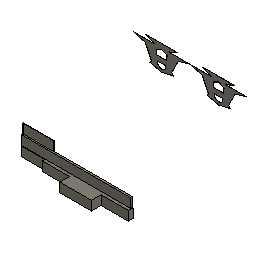
final drawing i hope v4 (Autodesk Fusion 360 design; units mm, degrees)
Autodesk Fusion 360 part; units mm, degrees
note: some values were not read from the file. Chosen so that the rebuilt part matches the saved one: which bodies a step acts on.
sketch "Sketch2" plane through (0, 0, 0) normal (0, 0, 1) x (1, 0, 0)
  line L0 (0, 0) -> (2438.4, 0)
  line L1 (2438.4, 0) -> (2438.4, 1219.2)
  line L2 (2438.4, 1219.2) -> (0, 1219.2)
  line L3 (0, 1219.2) -> (0, 0)
  line L4 (542.8322, 1080.4856) -> (1889.3565, 1080.4856)
  line L5 (1889.3565, 1080.4856) -> (1510.789, 917.945)
  line L6 (1510.789, 917.945) -> (2425.5578, 917.945)
  line L7 (2425.5578, 917.945) -> (1919.9959, 772.756)
  line L8 (1919.9959, 772.756) -> (1642.7832, 207.6244)
  line L9 (1642.7832, 207.6244) -> (1722.6773, 131.0438)
  line L10 (1722.6773, 131.0438) -> (1213.6665, 11.8411)
  line L11 (1211.4478, 868.4674) -> (1211.4478, 1080.4856)
  line L12 (1211.4478, 1080.4856) -> (1213.6665, 11.8411)
  line L13 (1213.6665, 11.8411) -> (1213.6665, 0)
  line L14 (1213.6665, 130.0044) -> (1361.4547, 188.3424)
  line L15 (1361.4547, 188.3424) -> (1391.2443, 341.6348)
  line L16 (1391.2443, 341.6348) -> (1212.9825, 341.2647)
  line L17 (1212.5359, 556.3863) -> (1420.4572, 556.818)
  line L18 (1420.4572, 556.818) -> (1446.4012, 750.0109)
  line L19 (1446.4012, 750.0109) -> (1211.4478, 868.4674)
  line L20 (1213.6665, 130.0044) -> (1361.4547, 188.3424)
  line L21 (1391.2443, 341.6348) -> (1361.4547, 188.3424)
  line L22 (1212.9825, 341.2647) -> (1391.2443, 341.6348)
  line L23 (1215.082, 130.5632) -> (1213.4213, 129.9077)
  dimension "d1" = 2438.4
  dimension "d2" = 1219.2
  constraint horizontal L0
  constraint vertical L1
  constraint horizontal L2
  constraint vertical L3
  constraint coincident L0.start L3.end
  constraint horizontal L4
  constraint perpendicular L1 L6
  constraint coincident L4 L11.end
  constraint perpendicular L4 L11
  constraint coincident L0 L13.end
  constraint perpendicular L0 L13
  constraint coincident L12 L16.end
  constraint perpendicular L12 L16
  constraint coincident L12 L17.start
  constraint perpendicular L12 L17
  constraint coincident L14 L23.start
  constraint coincident L12 L23.end
  constraint parallel L14 L23
  measures "d1" distance of L0.start L0.end
  measures "d2" distance of L0.start L2.end
extrude "Extrude1" add sketch "Sketch2" along normal blind 3.175 contours L4 L5 L6 L7 L8 L9 L10 L12 L14 L15 L16 L17 L18 L19 L20 L21 L22 L23 makes body 1
extrude "Extrude2" add 1 faces at (1661.0788, 512.3995, 3.175) along direction (0, 0, 1) blind 3.175 on bodies 1 bodies 1
mirror "Mirror1" about plane through (1212.5359, 556.3863, 0) normal (-0.999998, -0.002076, 0) of bodies 1 merged
sketch "Sketch3" plane through (0, 0, 0) normal (0, 0, 1) x (1, 0, 0)
  line L0 (0, 0) -> (-609.6, 0)
  line L1 (-609.6, 0) -> (-609.6, 406.4)
  line L2 (-609.6, 406.4) -> (0, 406.4)
  line L3 (0, 406.4) -> (0, 0)
  dimension "d9" = 609.6
  dimension "d10" = 406.4
  constraint horizontal L0
  constraint vertical L1
  constraint horizontal L2
  constraint vertical L3
  constraint coincident L0.start L3.end
  measures "d9" distance of L0.start L0.end
  measures "d10" distance of L0.start L2.end
scale "Scale1" factor 0.25 about (1004.6146, 555.9546, 6.35) bodies 1
move_body "Move1" bodies 1 to x (1, 0, 0) y (0, 1, 0) z (0, 0, 1) at (-1360.9962, -410.5353, 0)
scale "Scale2" factor 0.99 about (-356.3816, 145.4193, 6.35) bodies 1
move_body "Move2" bodies 1 to x (0, -1, 0) y (1, 0, 0) z (0, 0, 1) at (-608.2009, -92.7478, 0)
scale "Scale3" factor 0.650517 about (-332.9602, 212.4425, 4.7784) bodies 1
move_body "Move3" bodies 1 to x (1, 0, 0) y (0, 1, 0) z (0, 0, 1) at (-97.2386, -6.7841, 0)
sketch "Sketch4" plane through (0, 0, 0) normal (0, 1, 0) x (1, 0, 0)
sketch "Sketch5" plane through (0, 0, 0) normal (0, 0, 1) x (1, 0, 0)
  line L0 (203.9021, 0) -> (788.7117, 0)
  line L1 (788.7117, 196.85) -> (203.9021, 196.85)
  line L2 (203.9021, 196.85) -> (203.9021, 0)
  line L3 (203.9021, 0) -> (288.0777, 0)
  line L4 (288.0777, 0) -> (288.0777, 196.85)
  line L5 (288.0777, 196.85) -> (203.9021, 196.85)
  line L6 (203.9021, 196.85) -> (203.9021, 0)
  line L7 (288.0777, 196.85) -> (305.8831, 196.85)
  line L8 (305.8831, 196.85) -> (305.8831, 0)
  line L9 (305.8831, 0) -> (288.0777, 0)
  line L10 (288.0777, 0) -> (288.0777, 196.85)
  line L11 (305.8831, 196.85) -> (407.2291, 196.85)
  line L12 (407.2291, 196.85) -> (407.2291, 0)
  line L13 (407.2291, 0) -> (305.8831, 0)
  line L14 (305.8831, 0) -> (305.8831, 196.85)
  line L15 (407.2291, 196.85) -> (491.9127, 196.85)
  line L16 (491.9127, 196.85) -> (491.9127, 0)
  line L17 (491.9127, 0) -> (407.2291, 0)
  line L18 (407.2291, 0) -> (407.2291, 196.85)
  line L19 (491.9127, 196.85) -> (639.1819, 196.85)
  line L20 (639.1819, 196.85) -> (639.1819, 0)
  line L21 (639.1819, 0) -> (491.9127, 0)
  line L22 (491.9127, 0) -> (491.9127, 196.85)
  line L23 (639.1819, 196.85) -> (706.7713, 196.85)
  line L24 (706.7713, 196.85) -> (706.7713, 0)
  line L25 (706.7713, 0) -> (639.1819, 0)
  line L26 (639.1819, 0) -> (639.1819, 196.85)
  line L27 (706.7713, 196.85) -> (732.1713, 196.85)
  line L28 (732.1713, 196.85) -> (732.1713, 0)
  line L29 (732.1713, 0) -> (706.7713, 0)
  line L30 (706.7713, 0) -> (706.7713, 196.85)
  line L31 (732.1713, 196.85) -> (757.3173, 196.85)
  line L32 (757.3173, 196.85) -> (757.3173, 0)
  line L33 (757.3173, 0) -> (732.1713, 0)
  line L34 (732.1713, 0) -> (732.1713, 196.85)
  line L35 (757.3173, 196.85) -> (788.7117, 196.85)
  line L36 (788.7117, 196.85) -> (788.7117, 0)
  line L37 (788.7117, 0) -> (757.3173, 0)
  line L38 (757.3173, 0) -> (757.3173, 196.85)
  line L39 (203.9021, 98.425) -> (788.7117, 98.425)
  dimension "d15" = 196.85
  dimension "d16" = 84.1756
  dimension "d17" = 17.8054
  dimension "d18" = 101.346
  dimension "d19" = 84.6836
  dimension "d20" = 147.2692
  dimension "d21" = 67.5894
  dimension "d22" = 25.4
  dimension "d23" = 25.146
  dimension "d24" = 31.3944
  constraint horizontal L0
  constraint horizontal L1
  constraint vertical L2
  constraint horizontal L3
  constraint vertical L4
  constraint horizontal L5
  constraint vertical L6
  constraint coincident L1 L4.end
  constraint horizontal L7
  constraint vertical L8
  constraint horizontal L9
  constraint vertical L10
  constraint horizontal L11
  constraint vertical L12
  constraint horizontal L13
  constraint vertical L14
  constraint horizontal L15
  constraint vertical L16
  constraint horizontal L17
  constraint vertical L18
  constraint coincident L0 L16.end
  constraint horizontal L19
  constraint vertical L20
  constraint horizontal L21
  constraint vertical L22
  constraint horizontal L23
  constraint vertical L24
  constraint horizontal L25
  constraint vertical L26
  constraint coincident L0 L24.end
  constraint horizontal L27
  constraint vertical L28
  constraint horizontal L29
  constraint vertical L30
  constraint coincident L0 L28.end
  constraint horizontal L31
  constraint vertical L32
  constraint horizontal L33
  constraint vertical L34
  constraint horizontal L35
  constraint vertical L36
  constraint horizontal L37
  constraint vertical L38
  constraint midpoint L2 L39.start
  constraint midpoint L36 L39.end
  measures "d15" distance of L0.start L1.end
  measures "d16" distance of L0.start L3.end
  measures "d17" distance of L4.end L7.end
  measures "d18" distance of L7.end L11.end
  measures "d19" distance of L11.end L15.end
  measures "d20" distance of L15.end L19.end
  measures "d21" distance of L19.end L23.end
  measures "d22" distance of L23.end L27.end
  measures "d23" distance of L27.end L31.end
  measures "d24" distance of L31.end L1.start
sketch "Sketch6" plane through (0, 0, 0) normal (0, 0, 1) x (1, 0, 0)
  line L0 (822.2364, 571.8843) -> (212.6364, 571.8843)
  line L1 (212.6364, 571.8843) -> (212.6364, 375.0343)
  line L2 (212.6364, 375.0343) -> (822.2364, 375.0343)
  line L3 (822.2364, 375.0343) -> (822.2364, 571.8843)
  line L4 (212.6364, 571.8843) -> (254.9274, 571.8843)
  line L5 (254.9274, 571.8843) -> (254.9274, 375.0343)
  line L6 (254.9274, 375.0343) -> (212.6364, 375.0343)
  line L7 (212.6364, 375.0343) -> (212.6364, 571.8843)
  line L8 (254.9274, 571.8843) -> (312.3314, 571.8843)
  line L9 (312.3314, 571.8843) -> (312.3314, 473.4593)
  line L10 (312.3314, 375.0343) -> (254.9274, 375.0343)
  line L11 (254.9274, 375.0343) -> (254.9274, 571.8843)
  line L12 (212.6364, 473.4593) -> (254.9274, 473.4593)
  line L13 (312.3314, 571.8843) -> (379.2858, 571.8843)
  line L14 (379.2858, 571.8843) -> (379.2858, 473.4593)
  line L15 (379.2858, 375.0343) -> (312.3314, 375.0343)
  line L16 (312.3314, 473.4593) -> (312.3314, 571.8843)
  line L17 (254.9274, 473.4593) -> (379.2858, 473.4593)
  line L18 (254.9274, 473.4593) -> (473.215, 473.4593)
  line L19 (473.215, 473.4593) -> (473.215, 375.0343)
  line L20 (473.215, 375.0343) -> (254.9274, 375.0343)
  line L21 (254.9274, 375.0343) -> (254.9274, 473.4593)
  dimension "d25" = 609.6
  dimension "d26" = 196.85
  dimension "d27" = 42.291
  dimension "d28" = 57.404
  dimension "d29" = 66.9544
  dimension "d30" = 218.2876
  constraint horizontal L0
  constraint vertical L1
  constraint horizontal L2
  constraint vertical L3
  constraint horizontal L4
  constraint vertical L5
  constraint horizontal L6
  constraint vertical L7
  constraint horizontal L8
  constraint vertical L9
  constraint horizontal L10
  constraint vertical L11
  constraint coincident L2 L10.start
  constraint midpoint L7 L12.start
  constraint midpoint L11 L12.end
  constraint perpendicular L11 L12
  constraint horizontal L13
  constraint vertical L14
  constraint horizontal L15
  constraint vertical L16
  constraint coincident L2 L15.start
  constraint coincident L17 L9.end
  constraint horizontal L18
  constraint vertical L19
  constraint horizontal L20
  constraint vertical L21
  measures "d25" distance of L0.start L0.end
  measures "d26" distance of L0.start L2.end
  measures "d27" distance of L0.end L4.end
  measures "d28" distance of L4.end L8.end
  measures "d29" distance of L8.end L13.end
  measures "d30" distance of L12.end L18.end
extrude "Extrude3" add sketch "Sketch6" along normal blind 3.175 separate body contours L2 L5 L10 L11 L15 L17 L18 L19 L20 L21 makes body 2
move_body "Move4" bodies 2 to x (1, 0, 0) y (0, 1, 0) z (0, 0, 1) at (-384.6431, 161.5704, 0)
move_body "Move5" bodies 2 to x (0, -1, 0) y (0, 0, 1) z (-1, 0, 0) at (-430.0903, 185.4213, -530.8446)
extrude "Extrude4" add sketch "Sketch6" along normal blind 3.175 separate body contours L0 L9 L13 L14 L16 L17 L18 makes body 3
move_body "Move6" bodies 3 to x (0, -1, 0) y (0, 0, 1) z (-1, 0, 0) at (-514.5757, 550.6973, -468.49)
extrude "Extrude5" add sketch "Sketch6" along normal blind 3.175 separate body contours L0 L5 L8 L9 L11 L16 L17 L18 makes body 4
move_body "Move7" bodies 4 to x (0, 1, 0) y (0, 0, -1) z (-1, 0, 0) at (-545.9307, -77.9718, 577.731)
extrude "Extrude6" add sketch "Sketch6" along normal blind 3.175 separate body contours L0 L1 L4 L5 L7 L11 L12 makes body 5
move_body "Move8" bodies 5 to x (0.5, -0.866025, 0) y (0, 0, 1) z (-0.866025, -0.5, 0) at (-590.0447, 429.1998, -467.7351)
move_body "Move9" bodies 5 to x (0.99863, -0.052336, 0) y (0.052336, 0.99863, 0) z (0, 0, 1) at (-10.4106, -25.2848, 0)
copy_body "CopyPasteBodies1" bodies 5 makes body 6
move_body "Move10" bodies 6 to x (-0.587785, 0.809017, 0) y (-0.809017, -0.587785, 0) z (0, 0, 1) at (-568.0051, 700.1132, 0)
extrude "Extrude7" add sketch "Sketch5" along normal blind 3.175 separate body contours L1 L32 L35 L36 L38 L39 makes body 7
move_body "Move11" bodies 7 to x (0.990268, -0.139173, 0) y (0, 0, -1) z (0.139173, 0.990268, 0) at (-1264.9245, 274.1917, 98.425)
move_body "Move12" bodies 7 to x (1, 0, 0) y (0, 1, 0) z (0, 0, 1) at (0, 0, 104.14)
copy_body "CopyPasteBodies2" bodies 7 makes body 8
move_body "Move13" bodies 8 to x (0.956305, 0.292372, 0) y (-0.292372, 0.956305, 0) z (0, 0, 1) at (26.9574, 228.0991, 0)
scale "Scale4" factor 0.8 about (-514.8682, 238.9524, 5.715) bodies 1 7 4 5 2 6 3 8
sketch "Sketch7" plane through (0, 0, 0) normal (0, 0, 1) x (1, 0, 0)
  line L0 (0, 0) -> (196.85, 0)
  line L1 (196.85, 0) -> (196.85, 609.6)
  line L2 (196.85, 609.6) -> (0, 609.6)
  line L3 (0, 609.6) -> (0, 0)
  line L4 (0, 0) -> (98.425, 0)
  line L5 (98.425, 0) -> (98.425, 596.9)
  line L6 (98.425, 596.9) -> (0, 596.9)
  line L7 (0, 596.9) -> (0, 0)
  line L8 (0, 596.9) -> (196.85, 596.9)
  line L9 (196.85, 596.9) -> (196.85, 0)
  line L10 (196.85, 0) -> (0, 0)
  line L11 (0, 0) -> (0, 596.9)
  dimension "d42" = 196.85
  dimension "d43" = 609.6
  dimension "d44" = 98.425
  dimension "d45" = 596.9
  constraint horizontal L0
  constraint vertical L1
  constraint horizontal L2
  constraint vertical L3
  constraint coincident L0.start L3.end
  constraint horizontal L4
  constraint vertical L5
  constraint horizontal L6
  constraint vertical L7
  constraint horizontal L8
  constraint vertical L9
  constraint horizontal L10
  constraint vertical L11
  measures "d42" distance of L0.start L0.end
  measures "d43" distance of L0.start L2.end
  measures "d44" distance of L0.start L4.end
  measures "d45" distance of L0.start L6.end
sketch "Sketch8" plane through (0, 0, 0) normal (0, 0, 1) x (1, 0, 0)
  line L0 (-854.4402, -1.7894) -> (-1464.0402, -1.7894)
  line L1 (-1464.0402, -1.7894) -> (-1464.0402, 404.6106)
  line L2 (-1464.0402, 404.6106) -> (-854.4402, 404.6106)
  line L3 (-854.4402, 404.6106) -> (-854.4402, -1.7894)
  line L4 (-854.4402, 404.6106) -> (-1017.3075, 404.6106)
  line L5 (-1017.3075, 404.6106) -> (-1017.3075, 306.1856)
  line L6 (-1017.3075, 306.1856) -> (-854.4402, 306.1856)
  line L7 (-854.4402, 306.1856) -> (-854.4402, 404.6106)
  dimension "d46" = 609.6
  dimension "d47" = 406.4
  dimension "d48" = 162.8673
  dimension "d49" = 98.425
  constraint horizontal L0
  constraint vertical L1
  constraint horizontal L2
  constraint vertical L3
  constraint horizontal L4
  constraint vertical L5
  constraint horizontal L6
  constraint vertical L7
  measures "d46" distance of L0.start L0.end
  measures "d47" distance of L0.start L2.end
  measures "d48" distance of L2.end L4.end
  measures "d49" distance of L2.end L6.end
move_body "Move14" bodies 1 to x (1, 0, 0) y (0, 1, 0) z (0, 0, 1) at (-411.614, -53.3151, 0)
scale "Scale5" factor 0.869565 about (-981.0371, 93.1545, 4.9657) bodies 1
move_body "Move15" bodies 1 to x (1, 0, 0) y (0, 1, 0) z (0, 0, 1) at (15.801, -12.4151, 0)
sketch "Sketch9" plane through (0, 0, 0) normal (0, 0, 1) x (1, 0, 0)
  line L0 (-852.6405, 515.8905) -> (-852.6405, 319.0405)
  line L1 (-852.6405, 319.0405) -> (-1462.2405, 319.0405)
  line L2 (-1462.2405, 319.0405) -> (-1462.2405, 515.8905)
  line L3 (-1462.2405, 515.8905) -> (-852.6405, 515.8905)
  line L4 (-852.6405, 515.8905) -> (-852.6405, 417.4655)
  line L5 (-852.6405, 417.4655) -> (-1426.8837, 417.4655)
  line L6 (-1426.8837, 417.4655) -> (-1426.8837, 515.8905)
  line L7 (-1426.8837, 515.8905) -> (-852.6405, 515.8905)
  line L8 (-852.6405, 417.4655) -> (-852.6405, 319.0405)
  line L9 (-852.6405, 319.0405) -> (-1294.3465, 319.0405)
  line L10 (-1294.3465, 319.0405) -> (-1294.3465, 417.4655)
  line L11 (-1294.3465, 417.4655) -> (-852.6405, 417.4655)
  line L12 (-1462.2405, 319.0405) -> (-1462.2405, 417.4655)
  line L13 (-1462.2405, 417.4655) -> (-1337.8821, 417.4655)
  line L14 (-1337.8821, 417.4655) -> (-1337.8821, 319.0405)
  line L15 (-1337.8821, 319.0405) -> (-1462.2405, 319.0405)
  dimension "d51" = 196.85
  dimension "d52" = 609.6
  dimension "d53" = 98.425
  dimension "d54" = 574.2432
  dimension "d55" = 441.706
  dimension "d56" = 98.425
  dimension "d57" = 124.3584
  measures "d51" distance of L0.start L0.end
  measures "d52" distance of L0.start L2.end
  measures "d53" distance of L0.start L4.end
  measures "d54" distance of L0.start L6.end
  measures "d55" distance of L4.end L10.end
  measures "d56" distance of L1.end L12.end
  measures "d57" distance of L1.end L14.end
extrude "Extrude8" add sketch "Sketch9" along normal blind 25.4 separate body contours L0 L3 L4 L5 L6 L7 L11 L13 makes body 9
extrude "Extrude9" add sketch "Sketch9" along normal blind 50.8 contours L0 L1 L5 L8 L9 L10 L11 bodies 9
extrude "Extrude10" add sketch "Sketch9" along normal blind 101.6 contours L2 L3 L6 L13 bodies 9
extrude "Extrude11" add sketch "Sketch9" along normal blind 254 contours L1 L2 L5 L12 L13 L14 L15 bodies 9
extrude "Extrude12" add sketch "Sketch9" along normal blind 127 contours L1 L5 L10 L14 bodies 9
extrude "Extrude13" add sketch "Sketch8" along normal blind 50.8 separate body contours L2 L3 L4 L5 L6 L7 makes body 10
move_body "Move16" bodies 1 to x (1, 0, 0) y (0, 1, 0) z (0, 0, 1) at (193.7591, 897.4021, 0)
move_body "Move17" bodies 10 to x (1, 0, 0) y (0, 1, 0) z (0, 0, 1) at (211.1862, 486.0667, 0)
move_body "Move18" bodies 10 to x (1, 0, 0) y (0, 1, 0) z (0, 0, 1) at (-212.9978, -222.8284, 0)
move_body "Move19" bodies 1 to x (0, 1, 0) y (-1, 0, 0) z (0, 0, 1) at (-203.2687, 1330.3414, 0)
copy_body "CopyPasteBodies3" bodies 1 makes body 11
copy_body "CopyPasteBodies4" bodies 1 makes body 12
sketch "Sketch10" plane through (0, 0, 50.8) normal (0, 0, 1) x (1, 0, 0)
  line L0 (-856.2517, 569.4239) -> (-856.2517, 667.8489)
  line L1 (-856.2517, 667.8489) -> (-1019.1191, 667.8489)
  line L2 (-1019.1191, 667.8489) -> (-1019.1191, 569.4239)
  line L3 (-1019.1191, 569.4239) -> (-856.2517, 569.4239)
  line L4 (-1019.1191, 667.8489) -> (-856.2517, 667.8489)
  line L5 (-856.2517, 667.8489) -> (-856.2517, 618.6364)
  line L6 (-856.2517, 618.6364) -> (-1019.1191, 618.6364)
  line L7 (-1019.1191, 618.6364) -> (-1019.1191, 667.8489)
  constraint horizontal L4
  constraint vertical L5
  constraint horizontal L6
  constraint vertical L7
  constraint midpoint L0 L5.end
  constraint coincident L1.end L2.start
sketch "Sketch11" plane through (0, 0, 25.4) normal (0, 0, 1) x (1, 0, 0)
  line L0 (-1426.8837, 417.4655) -> (-852.6405, 417.4655)
  line L1 (-852.6405, 417.4655) -> (-852.6405, 515.8905)
  line L2 (-852.6405, 515.8905) -> (-1426.8837, 515.8905)
  line L3 (-1426.8837, 515.8905) -> (-1426.8837, 417.4655)
extrude "Extrude14" cut sketch "Sketch10" against normal blind 127 contours L0 L1 L2 L4 L5 L6 L7 bodies 10
sketch "Sketch12" plane through (0, 0, 254) normal (0, 0, 1) x (1, 0, 0)
  line L0 (-1337.8821, 319.0405) -> (-1337.8821, 417.4655)
  line L1 (-1337.8821, 417.4655) -> (-1462.2405, 417.4655)
  line L2 (-1462.2405, 417.4655) -> (-1462.2405, 319.0405)
  line L3 (-1462.2405, 319.0405) -> (-1337.8821, 319.0405)
  line L4 (-1462.2405, 417.4655) -> (-828.9163, 417.4655)
  line L5 (-828.9163, 417.4655) -> (-828.9163, 368.253)
  line L6 (-828.9163, 368.253) -> (-1462.2405, 368.253)
  line L7 (-1462.2405, 368.253) -> (-1462.2405, 417.4655)
  constraint horizontal L4
  constraint vertical L5
  constraint horizontal L6
  constraint vertical L7
  constraint coincident L1.end L2.start
extrude "Extrude15" cut sketch "Sketch12" against normal blind 482.6 contours L0 L1 L2 L4 L6 L7 | L0 L4 L5 L6 bodies 9 makes body 13 at (-1420.7877, 368.253, 127)
sketch "Sketch13" plane through (0, 0, 101.6) normal (0, 0, 1) x (1, 0, 0)
  line L0 (-1462.2405, 515.8905) -> (-1462.2405, 417.4655)
  line L1 (-1462.2405, 417.4655) -> (-1426.8837, 417.4655)
  line L2 (-1426.8837, 417.4655) -> (-1426.8837, 515.8905)
  line L3 (-1426.8837, 515.8905) -> (-1462.2405, 515.8905)
  line L4 (-1462.2405, 515.8905) -> (-807.734, 515.8905)
  line L5 (-807.734, 515.8905) -> (-807.734, 466.678)
  line L6 (-807.734, 466.678) -> (-1462.2405, 466.678)
  line L7 (-1462.2405, 466.678) -> (-1462.2405, 515.8905)
  constraint horizontal L4
  constraint vertical L5
  constraint horizontal L6
  constraint vertical L7
  constraint coincident L0.start L3.end
extrude "Extrude16" cut sketch "Sketch13" against normal blind 152.4 contours L0 L2 L3 L4 L6 L7 | L2 L4 L5 L6 bodies 9
sketch "Sketch14" plane through (0, 0, 127) normal (0, 0, 1) x (1, 0, 0)
  line L0 (-1294.3465, 368.253) -> (-1337.8821, 368.253)
  line L1 (-1337.8821, 368.253) -> (-1337.8821, 319.0405)
  line L2 (-1337.8821, 319.0405) -> (-1294.3465, 319.0405)
  line L3 (-1294.3465, 319.0405) -> (-1294.3465, 368.253)
  line L4 (-1337.8821, 368.253) -> (-1294.3465, 368.253)
  line L5 (-1294.3465, 368.253) -> (-1294.3465, 319.0405)
  line L6 (-1294.3465, 319.0405) -> (-1337.8821, 319.0405)
  line L7 (-1337.8821, 319.0405) -> (-1337.8821, 368.253)
  constraint horizontal L4
  constraint vertical L5
  constraint horizontal L6
  constraint vertical L7
  constraint coincident L2.end L3.start
  constraint coincident L0.end L1.start
extrude "Extrude17" cut sketch "Sketch14" against normal blind 609.6 bodies 13 makes body 14 at (-1379.3349, 368.253, 84.6667)
extrude "Extrude18" cut 1 faces at (-1438.6693, 433.8697, 101.6) along direction (0, 0, -1) blind 330.2 on bodies 9 bodies 9
move_body "Move20" bodies 13 to x (1, 0, 0) y (0, 1, 0) z (0, 0, 1) at (-43.372, 0.0855, 0)
move_body "Move21" bodies 9 to x (1, 0, 0) y (0, 1, 0) z (0, 0, 1) at (-35.3957, -49.0636, 0)
move_body "Move22" bodies 10 to x (1, 0, 0) y (0, 1, 0) z (0, 0, 1) at (-443.7944, -151.5396, 0)
move_body "Move23" bodies 11 to x (1, 0, 0) y (0, 1, 0) z (0, 0, 1) at (279.4, 0, 0)
sketch "Sketch15" plane through (0, 0, 0) normal (0, 0, 1) x (1, 0, 0)
copy_body "CopyPasteBodies5" bodies 11 makes body 15
move_body "Move24" bodies 15 to x (1, 0, 0) y (0, 1, 0) z (0, 0, 1) at (-13.7866, 164.5197, 0)
scale "Scale6" factor 1.1 about (-959.2196, 641.4325, 5.6769) bodies 15 11
move_body "Move25" bodies 15 to x (1, 0, 0) y (0, 1, 0) z (0, 0, 1) at (-327.2013, -180.1445, 0)
ref_plane "WorkPlane1" through (-1400.0613, 343.6468, 533.4) normal (0, 0, 1) x (1, 0, 0)
sketch "Sketch16" plane through (-1400.0613, 343.6468, 533.4) normal (0, 0, 1) x (1, 0, 0)
  line L0 (-62.1817, -24.6049) -> (62.5074, -24.6049)
  line L1 (62.5074, -24.6049) -> (62.5074, 24.6076)
  line L2 (62.5074, 24.6076) -> (-62.1817, 24.6076)
  line L3 (-62.1817, 24.6076) -> (-62.1817, -24.6049)
  line L4 (62.5074, 24.6076) -> (504.4253, 24.6076)
  line L5 (504.4253, 24.6076) -> (504.4253, -24.6049)
  line L6 (504.4253, -24.6049) -> (62.5074, -24.6049)
  line L7 (62.5074, -24.6049) -> (62.5074, 24.6076)
  line L8 (-62.1817, 24.6076) -> (512.6316, 24.6076)
  line L9 (512.6316, 24.6076) -> (512.6316, 73.8201)
  line L10 (512.6316, 73.8201) -> (-62.1817, 73.8201)
  line L11 (-62.1817, 73.8201) -> (-62.1817, 24.6076)
  line L12 (-62.1817, 73.8201) -> (100.4242, 73.8201)
  line L13 (100.4242, 73.8201) -> (100.4242, 123.0326)
  line L14 (100.4242, 123.0326) -> (-62.1817, 123.0326)
  line L15 (-62.1817, 123.0326) -> (-62.1817, 73.8201)
  dimension "d82" = 49.2125
  dimension "d83" = 49.2125
  dimension "d84" = 49.2125
  constraint horizontal L0
  constraint vertical L1
  constraint horizontal L2
  constraint vertical L3
  constraint horizontal L4
  constraint vertical L5
  constraint horizontal L6
  constraint vertical L7
  constraint horizontal L8
  constraint vertical L9
  constraint horizontal L10
  constraint vertical L11
  constraint horizontal L12
  constraint vertical L13
  constraint horizontal L14
  constraint vertical L15
  measures "d82" distance of L0.start L2.end
  measures "d83" distance of L2.end L10.end
  measures "d84" distance of L10.end L14.end
extrude "Extrude19" add sketch "Sketch16" along normal blind 2.54 separate body contours L10 L12 L13 L14 L15 makes body 16
extrude "Extrude20" add sketch "Sketch16" along normal blind 10.16 contours L2 L4 L8 L9 L10 L11 L12 bodies 16
extrude "Extrude21" add sketch "Sketch16" along normal blind 12.7 contours L0 L1 L2 L3 L7 L8 bodies 16
extrude "Extrude22" add sketch "Sketch16" along normal blind 25.4 contours L1 L4 L5 L6 L7 L8 bodies 16
move_body "Move26" bodies 15 to x (1, 0, 0) y (0, 1, 0) z (0, 0, 1) at (41.5198, -1.5382, 0)
sketch "Sketch17" plane through (0, 0, 558.8) normal (0, 0, 1) x (1, 0, 0)
  line L0 (-1337.5539, 319.0419) -> (-895.6361, 319.0419)
  line L1 (-895.6361, 319.0419) -> (-895.6361, 368.2544)
  line L2 (-895.6361, 368.2544) -> (-1337.5539, 368.2544)
  line L3 (-1337.5539, 368.2544) -> (-1337.5539, 319.0419)
  line L4 (-1116.595, 368.2544) -> (-1200.1102, 368.2544)
  line L5 (-1200.1102, 368.2544) -> (-1200.1102, 319.0419)
  line L6 (-1200.1102, 319.0419) -> (-1116.595, 319.0419)
  line L7 (-1116.595, 319.0419) -> (-1116.595, 368.2544)
  line L8 (-1200.1102, 368.2544) -> (-1033.0798, 368.2544)
  line L9 (-1033.0798, 368.2544) -> (-1033.0798, 319.0419)
  line L10 (-1033.0798, 319.0419) -> (-1200.1102, 319.0419)
  line L11 (-1200.1102, 319.0419) -> (-1200.1102, 368.2544)
  dimension "d93" = 83.5152
  dimension "d94" = 167.0304
  constraint horizontal L4
  constraint vertical L5
  constraint horizontal L6
  constraint vertical L7
  constraint midpoint L2 L4.start
  constraint horizontal L8
  constraint vertical L9
  constraint horizontal L10
  constraint vertical L11
  constraint coincident L0 L9.end
  measures "d93" distance of L4.start L4.end
  measures "d94" distance of L4.end L8.end
extrude "Extrude23" add 1 faces at (-895.6361, 335.4461, 545.2533) along direction (1, 0, 0) blind 12.7 on bodies 16 bodies 16
sketch "Sketch18" plane through (0, 0, 558.8) normal (0, 0, 1) x (1, 0, 0)
  line L0 (-1337.5539, 319.0419) -> (-882.9361, 319.0419)
  line L1 (-882.9361, 319.0419) -> (-882.9361, 368.2544)
  line L2 (-882.9361, 368.2544) -> (-1337.5539, 368.2544)
  line L3 (-1337.5539, 368.2544) -> (-1337.5539, 319.0419)
  line L4 (-1110.245, 368.2544) -> (-1193.7602, 368.2544)
  line L5 (-1193.7602, 368.2544) -> (-1193.7602, 319.0419)
  line L6 (-1193.7602, 319.0419) -> (-1110.245, 319.0419)
  line L7 (-1110.245, 319.0419) -> (-1110.245, 368.2544)
  line L8 (-1193.7602, 368.2544) -> (-1026.7298, 368.2544)
  line L9 (-1026.7298, 368.2544) -> (-1026.7298, 319.0419)
  line L10 (-1026.7298, 319.0419) -> (-1193.7602, 319.0419)
  line L11 (-1193.7602, 319.0419) -> (-1193.7602, 368.2544)
  dimension "d97" = 83.5152
  dimension "d98" = 167.0304
  constraint horizontal L4
  constraint vertical L5
  constraint horizontal L6
  constraint vertical L7
  constraint midpoint L2 L4.start
  constraint horizontal L8
  constraint vertical L9
  constraint horizontal L10
  constraint vertical L11
  measures "d97" distance of L4.start L4.end
  measures "d98" distance of L4.end L8.end
extrude "Extrude24" add sketch "Sketch18" along normal blind 50.8 contours L0 L2 L4 L5 L6 L7 L8 L10 L11 | L0 L2 L7 L8 L9 L10 bodies 16
hidden bodies 1 2 3 4 5 6 7 8 9 10 12 13 14
equation "d3 = ( 1 / 8 ) * 1 in"
equation "d5 = ( 1 / 8 ) * 1 in"
equation "d15 = 7 in + ( ( 3 / 4 ) * 1 in )"
equation "d26 = 7 in + ( ( 3 / 4 ) * 1 in )"
equation "d31 = ( 1 / 8 ) * 1 in"
equation "d33 = ( 1 / 8 ) * 1 in"
equation "d35 = ( 1 / 8 ) * 1 in"
equation "d37 = ( 1 / 8 ) * 1 in"
equation "d39 = ( 1 / 8 ) * 1 in"
equation "d44 = ( 7.75 / 2 ) * 1 in"
equation "d45 = ( 47 / 2 ) * 1 in"
equation "d50 = 40 / 46"
equation "d53 = ( 7.75 / 2 ) * 1 in"
equation "d56 = ( 7.75 / 2 ) * 1 in"
equation "d82 = ( 7.75 / 4 ) * 1 in"
equation "d83 = ( 7.75 / 4 ) * 1 in"
equation "d84 = ( 7.75 / 4 ) * 1 in"
equation "d93 = ( 6.576 / 2 ) * 1 in"
equation "d97 = ( 6.576 / 2 ) * 1 in"
named bodies: "h 2", "h 1"
